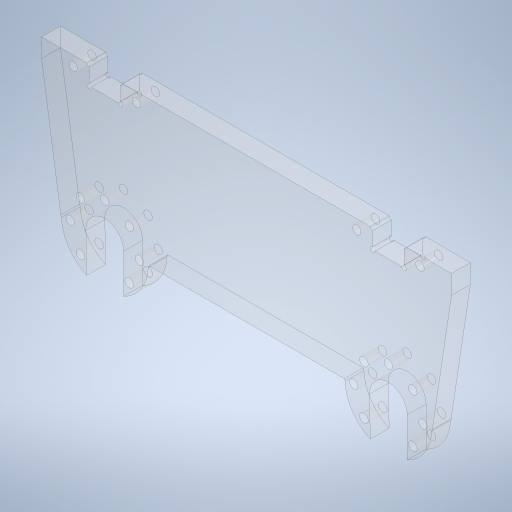
# Autodesk Inventor part: frame_pelvis_to_waist1
Saved by Autodesk Inventor 2024 (Build 280153000, 153)
## iProperties
Created: 2024-09-07
Part Number: frame_pelvis_to_waist1
Material: PMMA 플라스틱
Document SubType Name: Modeling
Designer: jmha0
Density: 1.188 g/cm^3
Appearance: 폴리카보네이트 - 선명
Author: jmha0
Autodesk Inventor part; units mm, degrees
ref_plane "YZ Plane" through (0, 0, 0) normal (1, 0, 0) x (0, 1, 0)
ref_plane "XZ Plane" through (0, 0, 0) normal (0, 1, 0) x (-1, 0, 0)
ref_plane "XY Plane" through (0, 0, 0) normal (0, 0, 1) x (1, 0, 0)
sketch "스케치1" plane through (0, 0, 0) normal (0, 0, 1) x (1, 0, 0)
  circle A0 centre (74.735, -11.0639) radius 1.35
  circle A1 centre (71.5132, -3.2858) radius 1.35
  circle A2 centre (55.9568, -3.2858) radius 1.35
  circle A3 centre (52.735, -11.0639) radius 1.35
  circle A4 centre (-18.6868, -3.2858) radius 1.35
  circle A5 centre (-15.465, -11.0639) radius 1.35
  circle A6 centre (-34.2432, -3.2858) radius 1.35
  circle A7 centre (-37.465, -11.0639) radius 1.35
  circle A8 centre (-26.465, -0.0639) radius 1.35
  circle A9 centre (63.735, -0.0639) radius 1.35
  line L0 (83.835, 28.9361) -> (83.835, 34.9361)
  line L1 (-46.565, 34.9361) -> (83.835, 34.9361)
  line L2 (-46.565, 28.9361) -> (-46.565, 34.9361)
  line L3 (-46.565, 28.9361) -> (-40.465, -11.0639)
  arc A10 (-40.465, -11.0639) -> (-33.915, -11.0639) centre (-37.19, -10.2275) ccw
  arc A11 (-19.015, -11.0639) -> (-33.915, -11.0639) centre (-26.465, -11.0639) ccw
  arc A12 (-19.015, -11.0639) -> (-12.465, -11.0639) centre (-15.74, -10.2126) ccw
  line L4 (-12.465, -11.0639) -> (49.735, -11.0639)
  arc A13 (49.735, -11.0639) -> (56.285, -11.0639) centre (53.01, -10.2275) ccw
  arc A14 (71.185, -11.0639) -> (56.285, -11.0639) centre (63.735, -11.0639) ccw
  arc A15 (71.185, -11.0639) -> (77.735, -11.0639) centre (74.46, -10.2126) ccw
  line L5 (77.735, -11.0639) -> (83.835, 28.9361)
  line L6 (-46.565, 28.9361) -> (83.835, 28.9361)
  circle A16 centre (-36.515, 31.9361) radius 1.35
  circle A17 centre (-16.415, 31.9361) radius 1.35
  circle A18 centre (73.785, 31.9361) radius 1.35
  circle A19 centre (53.685, 31.9361) radius 1.35
  point P0 (0, 0)
  point P1 (70.4566, 28.9361)
  dimension "d0" = 130.4
  dimension "d9" = 2.7
  dimension "d10" = 2.7
  dimension "d13" = 2.7
  dimension "d14" = 2.7
  dimension "d15" = 46
  constraints: 20 centre point, 14 end point, 12 point on circle, 1 horizontal
  measures "d0" distance of L1.start L0.end
  measures "d9" diameter of A16
  measures "d10" diameter of A17
  measures "d13" diameter of A18
  measures "d14" diameter of A19
  measures "d15" distance from line of A11.centre L1
extrude "돌출1" add sketch "스케치1" along normal blind 6
sketch "스케치2" plane through (0, 0, 6) normal (0, 0, 1) x (1, 0, 0)
  line L0 (83.835, 34.9361) -> (-46.565, 34.9361) projected
  line L1 (-46.565, 34.9361) -> (-46.565, 28.9361) projected
  line L2 (-46.565, 28.9361) -> (-40.465, -11.0639) projected
  arc A0 (-40.465, -11.0639) -> (-33.915, -11.0639) centre (-37.19, -10.2275) ccw projected
  arc A1 (-19.015, -11.0639) -> (-33.915, -11.0639) centre (-26.465, -11.0639) ccw projected
  arc A2 (-19.015, -11.0639) -> (-12.465, -11.0639) centre (-15.74, -10.2126) ccw projected
  line L3 (-12.465, -11.0639) -> (49.735, -11.0639) projected
  arc A3 (49.735, -11.0639) -> (56.285, -11.0639) centre (53.01, -10.2275) ccw projected
  arc A4 (71.185, -11.0639) -> (56.285, -11.0639) centre (63.735, -11.0639) ccw projected
  arc A5 (71.185, -11.0639) -> (77.735, -11.0639) centre (74.46, -10.2126) ccw projected
  line L4 (77.735, -11.0639) -> (83.835, 28.9361) projected
  line L5 (83.835, 28.9361) -> (83.835, 34.9361) projected
  circle A6 centre (74.735, -11.0639) radius 1.35 projected
  circle A7 centre (71.5132, -3.2858) radius 1.35 projected
  circle A8 centre (52.735, -11.0639) radius 1.35 projected
  circle A9 centre (55.9568, -3.2858) radius 1.35 projected
  circle A10 centre (-15.465, -11.0639) radius 1.35 projected
  circle A11 centre (-18.6868, -3.2858) radius 1.35 projected
  circle A12 centre (-37.465, -11.0639) radius 1.35 projected
  circle A13 centre (-34.2432, -3.2858) radius 1.35 projected
  circle A14 centre (-26.465, -0.0639) radius 1.35 projected
  circle A15 centre (63.735, -0.0639) radius 1.35 projected
  circle A16 centre (-36.515, 31.9361) radius 1.35 projected
  circle A17 centre (-16.415, 31.9361) radius 1.35 projected
  circle A18 centre (73.785, 31.9361) radius 1.35 projected
  circle A19 centre (53.685, 31.9361) radius 1.35 projected
  line L6 (-31.465, 28.9361) -> (-31.465, 34.9361)
  line L7 (-31.465, 34.9361) -> (-21.465, 34.9361)
  line L8 (-21.465, 34.9361) -> (-21.465, 28.9361)
  line L9 (-21.465, 28.9361) -> (-31.465, 28.9361)
  line L10 (-31.465, 28.9361) -> (-21.465, 34.9361) construction
  line L11 (-31.465, 34.9361) -> (-21.465, 28.9361) construction
  line L12 (58.735, 28.9361) -> (58.735, 34.9361)
  line L13 (58.735, 34.9361) -> (68.735, 34.9361)
  line L14 (68.735, 34.9361) -> (68.735, 28.9361)
  line L15 (68.735, 28.9361) -> (58.735, 28.9361)
  line L16 (58.735, 28.9361) -> (68.735, 34.9361) construction
  line L17 (58.735, 34.9361) -> (68.735, 28.9361) construction
  point P0 (0, 0)
  point P1 (-26.465, 31.9361)
  point P2 (63.735, 31.9361)
  dimension "d16" = 10
  dimension "d17" = 10
  constraints: 24 end point, 4 midpoint, 4 parallel, 4 perpendicular
  measures "d16" distance of L6.end L7.end
  measures "d17" distance of L12.end L13.end
extrude "돌출2" cut sketch "스케치2" against normal blind 10 contours L14 L15 L12 L0 | L8 L9 L6 L0
sketch "스케치3" plane through (0, 0, 6) normal (0, 0, 1) x (1, 0, 0)
  line L0 (58.735, 28.9361) -> (58.735, 34.9361) projected
  line L1 (58.735, 34.9361) -> (-21.465, 34.9361) projected
  line L2 (-21.465, 34.9361) -> (-21.465, 28.9361) projected
  line L3 (-21.465, 28.9361) -> (-31.465, 28.9361) projected
  line L4 (-31.465, 28.9361) -> (-31.465, 34.9361) projected
  line L5 (-31.465, 34.9361) -> (-46.565, 34.9361) projected
  line L6 (-46.565, 34.9361) -> (-46.565, 28.9361) projected
  line L7 (-46.565, 28.9361) -> (-40.465, -11.0639) projected
  arc A0 (-40.465, -11.0639) -> (-33.915, -11.0639) centre (-37.19, -10.2275) ccw projected
  arc A1 (-19.015, -11.0639) -> (-33.915, -11.0639) centre (-26.465, -11.0639) ccw projected
  arc A2 (-19.015, -11.0639) -> (-12.465, -11.0639) centre (-15.74, -10.2126) ccw projected
  line L8 (-12.465, -11.0639) -> (49.735, -11.0639) projected
  arc A3 (49.735, -11.0639) -> (56.285, -11.0639) centre (53.01, -10.2275) ccw projected
  arc A4 (71.185, -11.0639) -> (56.285, -11.0639) centre (63.735, -11.0639) ccw projected
  arc A5 (71.185, -11.0639) -> (77.735, -11.0639) centre (74.46, -10.2126) ccw projected
  line L9 (77.735, -11.0639) -> (83.835, 28.9361) projected
  line L10 (83.835, 28.9361) -> (83.835, 34.9361) projected
  line L11 (83.835, 34.9361) -> (68.735, 34.9361) projected
  line L12 (68.735, 34.9361) -> (68.735, 28.9361) projected
  line L13 (68.735, 28.9361) -> (58.735, 28.9361) projected
  circle A6 centre (74.735, -11.0639) radius 1.35 projected
  circle A7 centre (71.5132, -3.2858) radius 1.35 projected
  circle A8 centre (52.735, -11.0639) radius 1.35 projected
  circle A9 centre (55.9568, -3.2858) radius 1.35 projected
  circle A10 centre (-15.465, -11.0639) radius 1.35 projected
  circle A11 centre (-18.6868, -3.2858) radius 1.35 projected
  circle A12 centre (-37.465, -11.0639) radius 1.35 projected
  circle A13 centre (-34.2432, -3.2858) radius 1.35 projected
  circle A14 centre (-26.465, -0.0639) radius 1.35 projected
  circle A15 centre (63.735, -0.0639) radius 1.35 projected
  circle A16 centre (-36.515, 31.9361) radius 1.35 projected
  circle A17 centre (-16.415, 31.9361) radius 1.35 projected
  circle A18 centre (73.785, 31.9361) radius 1.35 projected
  circle A19 centre (53.685, 31.9361) radius 1.35 projected
  circle A20 centre (-31.465, 28.9361) radius 0.75
  circle A21 centre (-21.465, 28.9361) radius 0.75
  circle A22 centre (-31.465, 34.9361) radius 0.75
  circle A23 centre (-21.465, 34.9361) radius 0.75
  circle A24 centre (58.735, 28.9361) radius 0.75
  line L14 (58.735, 34.9361) -> (58.735, 28.9361) projected
  circle A25 centre (58.735, 34.9361) radius 0.75
  circle A26 centre (68.735, 34.9361) radius 0.75
  circle A27 centre (68.735, 28.9361) radius 0.75
  point P0 (0, 0)
  dimension "d20" = 1.5
  dimension "d21" = 1.5
  dimension "d22" = 1.5
  dimension "d23" = 1.5
  dimension "d24" = 1.5
  dimension "d25" = 1.5
  dimension "d26" = 1.5
  dimension "d27" = 1.5
  constraints: 8 centre point, 8 coincident
  measures "d20" diameter of A20
  measures "d21" diameter of A21
  measures "d22" diameter of A22
  measures "d23" diameter of A23
  measures "d24" diameter of A24
  measures "d25" diameter of A25
  measures "d26" diameter of A26
  measures "d27" diameter of A27
extrude "돌출3" cut sketch "스케치3" against normal blind 10 contours L13 A24 L0 | L0 A24 L13 | A25 L1 L0 | L0 L1 A25 | A27 L12 L13 | L13 L12 A27 | A23 L2 L1 | L1 L2 A23 | A26 L11 L12 | L12 L11 A26 | A21 L3 L2 | L2 L3 A21 | A20 L4 L3 | L3 L4 A20 | A22 L5 L4 | L4 L5 A22
sketch "스케치4" plane through (0, 0, 6) normal (0, 0, 1) x (1, 0, 0)
  line L0 (57.985, 34.9361) -> (-20.715, 34.9361) projected
  line L1 (57.985, 34.9361) -> (-20.715, 34.9361) projected
  line L2 (57.985, 34.9361) -> (-20.715, 34.9361) projected
  line L3 (57.985, 34.9361) -> (-20.715, 34.9361) projected
  line L4 (-12.465, -11.0639) -> (49.735, -11.0639) projected
  line L5 (-12.465, -11.0639) -> (49.735, -11.0639) projected
  line L6 (-12.465, -11.0639) -> (49.735, -11.0639) projected
  line L7 (-12.465, -11.0639) -> (49.735, -11.0639) projected
  arc A0 (-21.465, 34.1861) -> (-20.715, 34.9361) centre (-21.465, 34.9361) ccw projected
  line L8 (-21.465, 34.1861) -> (-21.465, 29.6861) projected
  arc A1 (-22.215, 28.9361) -> (-21.465, 29.6861) centre (-21.465, 28.9361) ccw projected
  line L9 (-22.215, 28.9361) -> (-30.715, 28.9361) projected
  arc A2 (-31.465, 29.6861) -> (-30.715, 28.9361) centre (-31.465, 28.9361) ccw projected
  line L10 (-31.465, 29.6861) -> (-31.465, 34.1861) projected
  arc A3 (-32.215, 34.9361) -> (-31.465, 34.1861) centre (-31.465, 34.9361) ccw projected
  line L11 (-32.215, 34.9361) -> (-46.565, 34.9361) projected
  line L12 (-46.565, 34.9361) -> (-46.565, 28.9361) projected
  line L13 (-46.565, 28.9361) -> (-40.465, -11.0639) projected
  arc A4 (-40.465, -11.0639) -> (-33.915, -11.0639) centre (-37.19, -10.2275) ccw projected
  arc A5 (-19.015, -11.0639) -> (-33.915, -11.0639) centre (-26.465, -11.0639) ccw projected
  arc A6 (-19.015, -11.0639) -> (-12.465, -11.0639) centre (-15.74, -10.2126) ccw projected
  line L14 (-12.465, -11.0639) -> (49.735, -11.0639) projected
  arc A7 (49.735, -11.0639) -> (56.285, -11.0639) centre (53.01, -10.2275) ccw projected
  arc A8 (71.185, -11.0639) -> (56.285, -11.0639) centre (63.735, -11.0639) ccw projected
  arc A9 (71.185, -11.0639) -> (77.735, -11.0639) centre (74.46, -10.2126) ccw projected
  line L15 (77.735, -11.0639) -> (83.835, 28.9361) projected
  line L16 (83.835, 28.9361) -> (83.835, 34.9361) projected
  line L17 (83.835, 34.9361) -> (69.485, 34.9361) projected
  arc A10 (68.735, 34.1861) -> (69.485, 34.9361) centre (68.735, 34.9361) ccw projected
  line L18 (68.735, 34.1861) -> (68.735, 29.6861) projected
  arc A11 (67.985, 28.9361) -> (68.735, 29.6861) centre (68.735, 28.9361) ccw projected
  line L19 (67.985, 28.9361) -> (59.485, 28.9361) projected
  arc A12 (58.735, 29.6861) -> (59.485, 28.9361) centre (58.735, 28.9361) ccw projected
  line L20 (58.735, 29.6861) -> (58.735, 34.1861) projected
  arc A13 (57.985, 34.9361) -> (58.735, 34.1861) centre (58.735, 34.9361) ccw projected
  line L21 (57.985, 34.9361) -> (-20.715, 34.9361) projected
  circle A14 centre (74.735, -11.0639) radius 1.35 projected
  circle A15 centre (71.5132, -3.2858) radius 1.35 projected
  circle A16 centre (52.735, -11.0639) radius 1.35 projected
  circle A17 centre (55.9568, -3.2858) radius 1.35 projected
  circle A18 centre (-15.465, -11.0639) radius 1.35 projected
  circle A19 centre (-18.6868, -3.2858) radius 1.35 projected
  circle A20 centre (-37.465, -11.0639) radius 1.35 projected
  circle A21 centre (-34.2432, -3.2858) radius 1.35 projected
  circle A22 centre (-26.465, -0.0639) radius 1.35 projected
  circle A23 centre (63.735, -0.0639) radius 1.35 projected
  circle A24 centre (-36.515, 31.9361) radius 1.35 projected
  circle A25 centre (-16.415, 31.9361) radius 1.35 projected
  circle A26 centre (73.785, 31.9361) radius 1.35 projected
  circle A27 centre (53.685, 31.9361) radius 1.35 projected
  circle A28 centre (74.735, -11.0639) radius 1.35 projected
  circle A29 centre (71.5132, -3.2858) radius 1.35 projected
  circle A30 centre (52.735, -11.0639) radius 1.35 projected
  circle A31 centre (55.9568, -3.2858) radius 1.35 projected
  circle A32 centre (-15.465, -11.0639) radius 1.35 projected
  circle A33 centre (-18.6868, -3.2858) radius 1.35 projected
  circle A34 centre (-37.465, -11.0639) radius 1.35 projected
  circle A35 centre (-34.2432, -3.2858) radius 1.35 projected
  circle A36 centre (-26.465, -0.0639) radius 1.35 projected
  circle A37 centre (63.735, -0.0639) radius 1.35 projected
  circle A38 centre (-36.515, 31.9361) radius 1.35 projected
  circle A39 centre (-16.415, 31.9361) radius 1.35 projected
  circle A40 centre (73.785, 31.9361) radius 1.35 projected
  circle A41 centre (53.685, 31.9361) radius 1.35 projected
  arc A42 (-21.465, 34.1861) -> (-20.715, 34.9361) centre (-21.465, 34.9361) ccw projected
  line L22 (57.985, 34.9361) -> (-20.715, 34.9361) projected
  arc A43 (57.985, 34.9361) -> (58.735, 34.1861) centre (58.735, 34.9361) ccw projected
  line L23 (58.735, 34.1861) -> (58.735, 29.6861) projected
  arc A44 (58.735, 29.6861) -> (59.485, 28.9361) centre (58.735, 28.9361) ccw projected
  line L24 (59.485, 28.9361) -> (67.985, 28.9361) projected
  arc A45 (67.985, 28.9361) -> (68.735, 29.6861) centre (68.735, 28.9361) ccw projected
  line L25 (68.735, 29.6861) -> (68.735, 34.1861) projected
  arc A46 (68.735, 34.1861) -> (69.485, 34.9361) centre (68.735, 34.9361) ccw projected
  line L26 (83.835, 34.9361) -> (69.485, 34.9361) projected
  line L27 (83.835, 28.9361) -> (83.835, 34.9361) projected
  line L28 (77.735, -11.0639) -> (83.835, 28.9361) projected
  arc A47 (71.185, -11.0639) -> (77.735, -11.0639) centre (74.46, -10.2126) ccw projected
  arc A48 (71.185, -11.0639) -> (56.285, -11.0639) centre (63.735, -11.0639) ccw projected
  arc A49 (49.735, -11.0639) -> (56.285, -11.0639) centre (53.01, -10.2275) ccw projected
  line L29 (-12.465, -11.0639) -> (49.735, -11.0639) projected
  arc A50 (-19.015, -11.0639) -> (-12.465, -11.0639) centre (-15.74, -10.2126) ccw projected
  arc A51 (-19.015, -11.0639) -> (-33.915, -11.0639) centre (-26.465, -11.0639) ccw projected
  arc A52 (-40.465, -11.0639) -> (-33.915, -11.0639) centre (-37.19, -10.2275) ccw projected
  line L30 (-46.565, 28.9361) -> (-40.465, -11.0639) projected
  line L31 (-46.565, 34.9361) -> (-46.565, 28.9361) projected
  line L32 (-32.215, 34.9361) -> (-46.565, 34.9361) projected
  arc A53 (-32.215, 34.9361) -> (-31.465, 34.1861) centre (-31.465, 34.9361) ccw projected
  line L33 (-31.465, 34.1861) -> (-31.465, 29.6861) projected
  arc A54 (-31.465, 29.6861) -> (-30.715, 28.9361) centre (-31.465, 28.9361) ccw projected
  line L34 (-30.715, 28.9361) -> (-22.215, 28.9361) projected
  arc A55 (-22.215, 28.9361) -> (-21.465, 29.6861) centre (-21.465, 28.9361) ccw projected
  line L35 (-21.465, 29.6861) -> (-21.465, 34.1861) projected
  arc A56 (57.985, 34.9361) -> (58.735, 34.1861) centre (58.735, 34.9361) ccw projected
  line L36 (58.735, 29.6861) -> (58.735, 34.1861) projected
  arc A57 (57.985, 34.9361) -> (58.735, 34.1861) centre (58.735, 34.9361) ccw projected
  arc A58 (57.985, 34.9361) -> (58.735, 34.1861) centre (58.735, 34.9361) ccw projected
  arc A59 (57.985, 34.9361) -> (58.735, 34.1861) centre (58.735, 34.9361) ccw projected
  line L37 (58.735, 34.1861) -> (58.735, 29.6861) projected
  line L38 (58.735, 29.6861) -> (58.735, 34.1861) projected
  line L39 (58.735, 34.1861) -> (58.735, 29.6861) projected
  arc A60 (58.735, 29.6861) -> (59.485, 28.9361) centre (58.735, 28.9361) ccw projected
  arc A61 (58.735, 29.6861) -> (59.485, 28.9361) centre (58.735, 28.9361) ccw projected
  arc A62 (58.735, 29.6861) -> (59.485, 28.9361) centre (58.735, 28.9361) ccw projected
  arc A63 (58.735, 29.6861) -> (59.485, 28.9361) centre (58.735, 28.9361) ccw projected
  circle A64 centre (55.9568, -3.2858) radius 1.35 projected
  circle A65 centre (55.9568, -3.2858) radius 1.35 projected
  circle A66 centre (55.9568, -3.2858) radius 1.35 projected
  arc A67 (68.735, 34.1861) -> (69.485, 34.9361) centre (68.735, 34.9361) ccw projected
  arc A68 (68.735, 34.1861) -> (69.485, 34.9361) centre (68.735, 34.9361) ccw projected
  arc A69 (67.985, 28.9361) -> (68.735, 29.6861) centre (68.735, 28.9361) ccw projected
  circle A70 centre (63.735, -0.0639) radius 1.35 projected
  circle A71 centre (63.735, -0.0639) radius 1.35 projected
  circle A72 centre (74.735, -11.0639) radius 1.35 projected
  arc A73 (-32.215, 34.9361) -> (-31.465, 34.1861) centre (-31.465, 34.9361) ccw projected
  circle A74 centre (71.5132, -3.2858) radius 1.35 projected
  arc A75 (67.985, 28.9361) -> (68.735, 29.6861) centre (68.735, 28.9361) ccw projected
  arc A76 (49.735, -11.0639) -> (56.285, -11.0639) centre (53.01, -10.2275) ccw projected
  arc A77 (49.735, -11.0639) -> (56.285, -11.0639) centre (53.01, -10.2275) ccw projected
  arc A78 (71.185, -11.0639) -> (56.285, -11.0639) centre (63.735, -11.0639) ccw projected
  arc A79 (71.185, -11.0639) -> (56.285, -11.0639) centre (63.735, -11.0639) ccw projected
  arc A80 (71.185, -11.0639) -> (56.285, -11.0639) centre (63.735, -11.0639) ccw projected
  arc A81 (71.185, -11.0639) -> (56.285, -11.0639) centre (63.735, -11.0639) ccw projected
  arc A82 (-22.215, 28.9361) -> (-21.465, 29.6861) centre (-21.465, 28.9361) ccw projected
  arc A83 (-22.215, 28.9361) -> (-21.465, 29.6861) centre (-21.465, 28.9361) ccw projected
  arc A84 (-32.215, 34.9361) -> (-31.465, 34.1861) centre (-31.465, 34.9361) ccw projected
  circle A85 centre (63.735, -0.0639) radius 1.35 projected
  circle A86 centre (55.9568, -3.2858) radius 1.35 projected
  arc A87 (-21.465, 34.1861) -> (-20.715, 34.9361) centre (-21.465, 34.9361) ccw projected
  arc A88 (-31.465, 29.6861) -> (-30.715, 28.9361) centre (-31.465, 28.9361) ccw projected
  arc A89 (-31.465, 29.6861) -> (-30.715, 28.9361) centre (-31.465, 28.9361) ccw projected
  line L40 (-31.465, 34.1861) -> (-31.465, 29.6861) projected
  arc A90 (-21.465, 34.1861) -> (-20.715, 34.9361) centre (-21.465, 34.9361) ccw projected
  circle A91 centre (52.735, -11.0639) radius 1.35 projected
  circle A92 centre (52.735, -11.0639) radius 1.35 projected
  circle A93 centre (52.735, -11.0639) radius 1.35 projected
  circle A94 centre (52.735, -11.0639) radius 1.35 projected
  circle A95 centre (-18.6868, -3.2858) radius 1.35 projected
  line L41 (-31.465, 29.6861) -> (-31.465, 34.1861) projected
  circle A96 centre (-16.415, 31.9361) radius 1.35 projected
  line L42 (67.985, 28.9361) -> (59.485, 28.9361) projected
  circle A97 centre (53.685, 31.9361) radius 1.35 projected
  circle A98 centre (53.685, 31.9361) radius 1.35 projected
  circle A99 centre (53.685, 31.9361) radius 1.35 projected
  line L43 (59.485, 28.9361) -> (67.985, 28.9361) projected
  line L44 (67.985, 28.9361) -> (59.485, 28.9361) projected
  circle A100 centre (53.685, 31.9361) radius 1.35 projected
  circle A101 centre (73.785, 31.9361) radius 1.35 projected
  line L45 (68.735, 29.6861) -> (68.735, 34.1861) projected
  line L46 (83.835, 34.9361) -> (69.485, 34.9361) projected
  line L47 (83.835, 28.9361) -> (83.835, 34.9361) projected
  line L48 (59.485, 28.9361) -> (67.985, 28.9361) projected
  circle A102 centre (-15.465, -11.0639) radius 1.35 projected
  circle A103 centre (-37.465, -11.0639) radius 1.35 projected
  arc A104 (-19.015, -11.0639) -> (-12.465, -11.0639) centre (-15.74, -10.2126) ccw projected
  arc A105 (-19.015, -11.0639) -> (-33.915, -11.0639) centre (-26.465, -11.0639) ccw projected
  arc A106 (71.185, -11.0639) -> (77.735, -11.0639) centre (74.46, -10.2126) ccw projected
  line L49 (77.735, -11.0639) -> (83.835, 28.9361) projected
  line L50 (77.735, -11.0639) -> (83.835, 28.9361) projected
  line L51 (77.735, -11.0639) -> (83.835, 28.9361) projected
  line L52 (77.735, -11.0639) -> (83.835, 28.9361) projected
  circle A107 centre (-34.2432, -3.2858) radius 1.35 projected
  circle A108 centre (-26.465, -0.0639) radius 1.35 projected
  circle A109 centre (-36.515, 31.9361) radius 1.35 projected
  line L53 (-21.465, 29.6861) -> (-21.465, 34.1861) projected
  arc A110 (-40.465, -11.0639) -> (-33.915, -11.0639) centre (-37.19, -10.2275) ccw projected
  line L54 (-46.565, 28.9361) -> (-40.465, -11.0639) projected
  line L55 (-46.565, 34.9361) -> (-46.565, 28.9361) projected
  line L56 (-32.215, 34.9361) -> (-46.565, 34.9361) projected
  line L57 (-30.715, 28.9361) -> (-22.215, 28.9361) projected
  arc A111 (49.735, -11.0639) -> (56.285, -11.0639) centre (53.01, -10.2275) ccw projected
  arc A112 (71.185, -11.0639) -> (77.735, -11.0639) centre (74.46, -10.2126) ccw projected
  arc A113 (71.185, -11.0639) -> (77.735, -11.0639) centre (74.46, -10.2126) ccw projected
  arc A114 (71.185, -11.0639) -> (77.735, -11.0639) centre (74.46, -10.2126) ccw projected
  circle A115 centre (74.735, -11.0639) radius 1.35 projected
  circle A116 centre (74.735, -11.0639) radius 1.35 projected
  circle A117 centre (74.735, -11.0639) radius 1.35 projected
  line L58 (-21.465, 34.1861) -> (-21.465, 29.6861) projected
  line L59 (-22.215, 28.9361) -> (-30.715, 28.9361) projected
  line L60 (-32.215, 34.9361) -> (-46.565, 34.9361) projected
  arc A118 (-19.015, -11.0639) -> (-33.915, -11.0639) centre (-26.465, -11.0639) ccw projected
  line L61 (-46.565, 34.9361) -> (-46.565, 28.9361) projected
  line L62 (-46.565, 28.9361) -> (-40.465, -11.0639) projected
  arc A119 (-40.465, -11.0639) -> (-33.915, -11.0639) centre (-37.19, -10.2275) ccw projected
  arc A120 (-19.015, -11.0639) -> (-12.465, -11.0639) centre (-15.74, -10.2126) ccw projected
  arc A121 (49.735, -11.0639) -> (56.285, -11.0639) centre (53.01, -10.2275) ccw projected
  arc A122 (67.985, 28.9361) -> (68.735, 29.6861) centre (68.735, 28.9361) ccw projected
  arc A123 (67.985, 28.9361) -> (68.735, 29.6861) centre (68.735, 28.9361) ccw projected
  circle A124 centre (73.785, 31.9361) radius 1.35 projected
  circle A125 centre (73.785, 31.9361) radius 1.35 projected
  circle A126 centre (73.785, 31.9361) radius 1.35 projected
  arc A127 (68.735, 34.1861) -> (69.485, 34.9361) centre (68.735, 34.9361) ccw projected
  arc A128 (68.735, 34.1861) -> (69.485, 34.9361) centre (68.735, 34.9361) ccw projected
  line L63 (68.735, 34.1861) -> (68.735, 29.6861) projected
  line L64 (83.835, 28.9361) -> (83.835, 34.9361) projected
  line L65 (83.835, 28.9361) -> (83.835, 34.9361) projected
  line L66 (83.835, 28.9361) -> (83.835, 34.9361) projected
  line L67 (83.835, 34.9361) -> (69.485, 34.9361) projected
  line L68 (83.835, 34.9361) -> (69.485, 34.9361) projected
  line L69 (83.835, 34.9361) -> (69.485, 34.9361) projected
  line L70 (68.735, 34.1861) -> (68.735, 29.6861) projected
  line L71 (68.735, 29.6861) -> (68.735, 34.1861) projected
  circle A129 centre (-15.465, -11.0639) radius 1.35 projected
  circle A130 centre (-18.6868, -3.2858) radius 1.35 projected
  circle A131 centre (-37.465, -11.0639) radius 1.35 projected
  circle A132 centre (-34.2432, -3.2858) radius 1.35 projected
  circle A133 centre (-26.465, -0.0639) radius 1.35 projected
  circle A134 centre (-36.515, 31.9361) radius 1.35 projected
  circle A135 centre (-16.415, 31.9361) radius 1.35 projected
  arc A136 (-21.465, 34.1861) -> (-20.715, 34.9361) centre (-21.465, 34.9361) ccw projected
  arc A137 (-21.465, 34.1861) -> (-20.715, 34.9361) centre (-21.465, 34.9361) ccw projected
  arc A138 (-31.465, 29.6861) -> (-30.715, 28.9361) centre (-31.465, 28.9361) ccw projected
  arc A139 (-31.465, 29.6861) -> (-30.715, 28.9361) centre (-31.465, 28.9361) ccw projected
  arc A140 (-32.215, 34.9361) -> (-31.465, 34.1861) centre (-31.465, 34.9361) ccw projected
  arc A141 (-32.215, 34.9361) -> (-31.465, 34.1861) centre (-31.465, 34.9361) ccw projected
  arc A142 (-22.215, 28.9361) -> (-21.465, 29.6861) centre (-21.465, 28.9361) ccw projected
  arc A143 (-22.215, 28.9361) -> (-21.465, 29.6861) centre (-21.465, 28.9361) ccw projected
  line L72 (-31.465, 34.1861) -> (-31.465, 29.6861) projected
  line L73 (-31.465, 29.6861) -> (-31.465, 34.1861) projected
  circle A144 centre (-15.465, -11.0639) radius 1.35 projected
  circle A145 centre (-15.465, -11.0639) radius 1.35 projected
  circle A146 centre (-16.415, 31.9361) radius 1.35 projected
  circle A147 centre (-16.415, 31.9361) radius 1.35 projected
  arc A148 (-19.015, -11.0639) -> (-12.465, -11.0639) centre (-15.74, -10.2126) ccw projected
  arc A149 (-19.015, -11.0639) -> (-12.465, -11.0639) centre (-15.74, -10.2126) ccw projected
  circle A150 centre (-18.6868, -3.2858) radius 1.35 projected
  circle A151 centre (-18.6868, -3.2858) radius 1.35 projected
  circle A152 centre (-26.465, -0.0639) radius 1.35 projected
  circle A153 centre (-26.465, -0.0639) radius 1.35 projected
  line L74 (-22.215, 28.9361) -> (-30.715, 28.9361) projected
  line L75 (-30.715, 28.9361) -> (-22.215, 28.9361) projected
  arc A154 (-19.015, -11.0639) -> (-33.915, -11.0639) centre (-26.465, -11.0639) ccw projected
  arc A155 (-19.015, -11.0639) -> (-33.915, -11.0639) centre (-26.465, -11.0639) ccw projected
  circle A156 centre (-34.2432, -3.2858) radius 1.35 projected
  circle A157 centre (-34.2432, -3.2858) radius 1.35 projected
  circle A158 centre (-36.515, 31.9361) radius 1.35 projected
  circle A159 centre (-36.515, 31.9361) radius 1.35 projected
  circle A160 centre (-37.465, -11.0639) radius 1.35 projected
  circle A161 centre (-37.465, -11.0639) radius 1.35 projected
  arc A162 (-40.465, -11.0639) -> (-33.915, -11.0639) centre (-37.19, -10.2275) ccw projected
  arc A163 (-40.465, -11.0639) -> (-33.915, -11.0639) centre (-37.19, -10.2275) ccw projected
  line L76 (-46.565, 28.9361) -> (-40.465, -11.0639) projected
  line L77 (-46.565, 28.9361) -> (-40.465, -11.0639) projected
  line L78 (-46.565, 34.9361) -> (-46.565, 28.9361) projected
  line L79 (-46.565, 34.9361) -> (-46.565, 28.9361) projected
  line L80 (-32.215, 34.9361) -> (-46.565, 34.9361) projected
  line L81 (-32.215, 34.9361) -> (-46.565, 34.9361) projected
  line L82 (-21.465, 29.6861) -> (-21.465, 34.1861) projected
  line L83 (-21.465, 34.1861) -> (-21.465, 29.6861) projected
  circle A164 centre (71.5132, -3.2858) radius 1.35 projected
  circle A165 centre (71.5132, -3.2858) radius 1.35 projected
  circle A166 centre (71.5132, -3.2858) radius 1.35 projected
  circle A167 centre (63.735, -0.0639) radius 1.35 projected
  circle A168 centre (-26.465, -11.0639) radius 13.8
  circle A169 centre (-26.465, -22.0639) radius 1.2813
  circle A170 centre (-34.2432, -18.8421) radius 1.2813
  circle A171 centre (-37.465, -11.0639) radius 1.2813
  circle A172 centre (-34.2432, -3.2858) radius 1.2813
  circle A173 centre (-26.465, -0.0639) radius 1.2813
  circle A174 centre (-18.6868, -3.2858) radius 1.2813
  circle A175 centre (-15.465, -11.0639) radius 1.2813
  circle A176 centre (-18.6868, -18.8421) radius 1.2813
  circle A177 centre (-26.465, -11.0639) radius 6
  line L84 (-32.465, -11.0639) -> (-32.215, -23.609)
  line L85 (-20.465, -11.0639) -> (-20.465, -23.4913)
  circle A178 centre (-18.6868, -18.8421) radius 1.3813
  circle A179 centre (-34.2432, -18.8421) radius 1.3813
  arc A180 (49.735, -11.0639) -> (56.285, -11.0639) centre (53.01, -10.2275) ccw
  arc A181 (71.185, -11.0639) -> (56.285, -11.0639) centre (63.735, -11.0639) ccw
  arc A182 (71.185, -11.0639) -> (77.735, -11.0639) centre (74.46, -10.2126) ccw
  circle A183 centre (74.735, -11.0639) radius 1.35
  circle A184 centre (71.5132, -3.2858) radius 1.35
  circle A185 centre (52.735, -11.0639) radius 1.35
  circle A186 centre (55.9568, -3.2858) radius 1.35
  circle A187 centre (63.735, -0.0639) radius 1.35
  circle A188 centre (74.735, -11.0639) radius 1.35
  circle A189 centre (71.5132, -3.2858) radius 1.35
  circle A190 centre (52.735, -11.0639) radius 1.35
  circle A191 centre (55.9568, -3.2858) radius 1.35
  circle A192 centre (63.735, -0.0639) radius 1.35
  arc A193 (71.185, -11.0639) -> (77.735, -11.0639) centre (74.46, -10.2126) ccw
  arc A194 (71.185, -11.0639) -> (56.285, -11.0639) centre (63.735, -11.0639) ccw
  arc A195 (49.735, -11.0639) -> (56.285, -11.0639) centre (53.01, -10.2275) ccw
  circle A196 centre (71.5132, -3.2858) radius 1.35
  circle A197 centre (74.735, -11.0639) radius 1.35
  circle A198 centre (52.735, -11.0639) radius 1.35
  arc A199 (71.185, -11.0639) -> (77.735, -11.0639) centre (74.46, -10.2126) ccw
  arc A200 (71.185, -11.0639) -> (56.285, -11.0639) centre (63.735, -11.0639) ccw
  circle A201 centre (55.9568, -3.2858) radius 1.35
  circle A202 centre (63.735, -0.0639) radius 1.35
  arc A203 (49.735, -11.0639) -> (56.285, -11.0639) centre (53.01, -10.2275) ccw
  arc A204 (71.185, -11.0639) -> (56.285, -11.0639) centre (63.735, -11.0639) ccw
  arc A205 (49.735, -11.0639) -> (56.285, -11.0639) centre (53.01, -10.2275) ccw
  arc A206 (71.185, -11.0639) -> (77.735, -11.0639) centre (74.46, -10.2126) ccw
  circle A207 centre (74.735, -11.0639) radius 1.35
  circle A208 centre (71.5132, -3.2858) radius 1.35
  circle A209 centre (52.735, -11.0639) radius 1.35
  circle A210 centre (55.9568, -3.2858) radius 1.35
  circle A211 centre (63.735, -0.0639) radius 1.35
  circle A212 centre (74.735, -11.0639) radius 1.35
  circle A213 centre (74.735, -11.0639) radius 1.35
  arc A214 (71.185, -11.0639) -> (77.735, -11.0639) centre (74.46, -10.2126) ccw
  arc A215 (71.185, -11.0639) -> (77.735, -11.0639) centre (74.46, -10.2126) ccw
  circle A216 centre (71.5132, -3.2858) radius 1.35
  circle A217 centre (71.5132, -3.2858) radius 1.35
  circle A218 centre (63.735, -0.0639) radius 1.35
  circle A219 centre (63.735, -0.0639) radius 1.35
  arc A220 (71.185, -11.0639) -> (56.285, -11.0639) centre (63.735, -11.0639) ccw
  arc A221 (71.185, -11.0639) -> (56.285, -11.0639) centre (63.735, -11.0639) ccw
  circle A222 centre (55.9568, -3.2858) radius 1.35
  circle A223 centre (55.9568, -3.2858) radius 1.35
  circle A224 centre (52.735, -11.0639) radius 1.35
  circle A225 centre (52.735, -11.0639) radius 1.35
  arc A226 (49.735, -11.0639) -> (56.285, -11.0639) centre (53.01, -10.2275) ccw
  arc A227 (49.735, -11.0639) -> (56.285, -11.0639) centre (53.01, -10.2275) ccw
  circle A228 centre (63.735, -11.0639) radius 13.8
  circle A229 centre (63.735, -22.0639) radius 1.2813
  circle A230 centre (55.9568, -18.8421) radius 1.2813
  circle A231 centre (52.735, -11.0639) radius 1.2813
  circle A232 centre (55.9568, -3.2858) radius 1.2813
  circle A233 centre (63.735, -0.0639) radius 1.2813
  circle A234 centre (71.5132, -3.2858) radius 1.2813
  circle A235 centre (74.735, -11.0639) radius 1.2813
  circle A236 centre (71.5132, -18.8421) radius 1.2813
  circle A237 centre (63.735, -11.0639) radius 6
  line L86 (57.735, -11.0639) -> (57.985, -23.609)
  line L87 (69.735, -11.0639) -> (69.735, -23.4913)
  circle A238 centre (71.5132, -18.8421) radius 1.3813
  circle A239 centre (55.9568, -18.8421) radius 1.3813
  point P0 (0, 0)
  point P1 (-26.465, -11.0639)
  point P2 (-12.6775, -11.6519)
  point P3 (-40.2522, -11.6587)
  point P4 (-32.4602, -11.303)
  point P5 (77.735, -11.0639)
  point P6 (77.735, -11.0639)
  point P7 (63.735, -11.0639)
  point P8 (77.5225, -11.6519)
  point P9 (49.9478, -11.6587)
  point P10 (57.7398, -11.303)
  dimension "d30" = 12
  dimension "d31" = 0.1
  dimension "d32" = 0.1
  dimension "d35" = 12
  dimension "d36" = 0.1
  dimension "d37" = 0.1
  constraints: 72 centre point, 44 point on circle, 8 end point, 2 tangent, 2 vertical, 3 other
  measures "d30" diameter of A177
  measures "d31" radial gap between concentric circles of A176 A178
  measures "d32" radial gap between concentric circles of A170 A179
  measures "d35" diameter of A237
  measures "d36" radial gap between concentric circles of A236 A238
  measures "d37" radial gap between concentric circles of A230 A239
extrude "돌출4" add sketch "스케치4" against normal blind 6 contours A228 L87 A237 L86 A7 A8 A9 | A4 A5 A6 A168 L85 A177 L84
